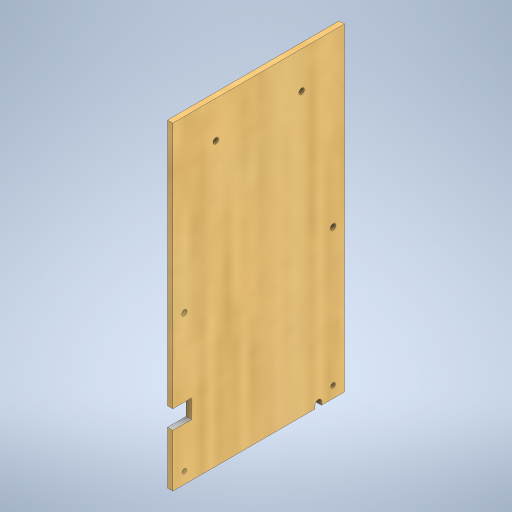
# Autodesk Inventor part: Panel2
Saved by Autodesk Inventor 2023 (Build 270158000, 158)
## iProperties
Created: 2022-12-03
Part Number: Panel2
Material: Genérico
Document SubType Name: Modeling
Designer: sergi
Density: 1 g/cm^3
Appearance: Valor por defecto
Author: sergi
Autodesk Inventor part; units mm, degrees
ref_plane "YZ Plane" through (0, 0, 0) normal (1, 0, 0) x (0, 1, 0)
ref_plane "XZ Plane" through (0, 0, 0) normal (0, 1, 0) x (-1, 0, 0)
ref_plane "XY Plane" through (0, 0, 0) normal (0, 0, 1) x (1, 0, 0)
sketch "Boceto1" plane through (0, 0, 0) normal (0, 1, 0) x (-1, 0, 0)
  line L0 (-1.5, -48.5) -> (1.5, -48.5)
  line L1 (1.5, -48.5) -> (1.5, 48.5)
  line L2 (1.5, 48.5) -> (-1.5, 48.5)
  line L3 (-1.5, 48.5) -> (-1.5, -48.5)
  line L4 (-1.5, -48.5) -> (1.5, 48.5) construction
  line L5 (1.5, -48.5) -> (-1.5, 48.5) construction
  point P0 (0, 0)
  dimension "d0" = 3
  dimension "d1" = 97
  constraints: 12 end point, 2 midpoint, 2 parallel, 1 horizontal, 1 perpendicular
  measures "d0" distance of L2.end L1.end
  measures "d1" distance of L1.end L0.end
extrude "Extrusión1" add sketch "Boceto1" along normal blind 180
sketch "Boceto2" plane through (-1.5, 0, -48.5) normal (-1, 0, 0) x (0, 0, 1)
  circle A0 centre (24.25, 159.25) radius 1.5 projected
  circle A1 centre (72.75, 159.25) radius 1.5 projected
  circle A2 centre (90.5, 84) radius 1.5 projected
  circle A3 centre (6.5, 84) radius 1.5 projected
  circle A4 centre (6.5, 6.5) radius 1.25 projected
  circle A5 centre (90.5, 6.5) radius 1.25 projected
  point P0 (48.5, 0)
extrude "Extrusión2" cut sketch "Boceto2" against normal through all
sketch "Boceto3" plane through (1.5, 0, 48.5) normal (1, 0, 0) x (0, 0, -1)
  line L0 (10.5, 26) -> (5.5, 26)
  line L1 (10.5, 44) -> (10.5, 26)
  line L2 (5.5, 44) -> (-0.0781, 44)
  line L3 (-0.0781, 26) -> (5.5, 26)
  line L4 (0, 0) -> (0, 180) projected
  line L5 (0, 44) -> (10.5, 44)
  line L6 (10.5, 44) -> (10.5, 26)
  line L7 (10.5, 26) -> (0, 26)
  line L8 (0, 26) -> (0, 44)
  line L9 (0, 35) -> (10.5, 35)
  line L10 (10.5, 29.75) -> (0, 29.75)
  line L11 (0, 29.75) -> (0, 40.25)
  line L12 (0, 40.25) -> (10.5, 40.25)
  line L13 (10.5, 40.25) -> (10.5, 29.75)
  line L14 (10.5, 29.75) -> (0, 40.25) construction
  line L15 (0, 29.75) -> (10.5, 40.25) construction
  point P0 (48.5, 0)
  point P1 (5.25, 35)
  point P2 (10.5, 40.25)
  point P3 (10.5, 29.75)
  dimension "d13" = 10.5
  constraints: 30 end point, 5 midpoint, 5 parallel, 4 horizontal, 3 point on line, 2 perpendicular
  measures "d13" distance of L10.end L11.end
extrude "Extrusión3" cut sketch "Boceto3" against normal through all contours L10 L4 L9 L1 | L9 L4 L12 L1
sketch "Boceto4" plane through (1.5, 0, 48.5) normal (1, 0, 0) x (0, 0, -1)
  line L0 (84, 0) -> (84, 13) projected
  line L1 (100, 0) -> (-3, 0) projected
  arc A0 (84, 1.85) -> (80.3, 1.85) centre (82.15, 1.85) ccw
  line L2 (0, 0) -> (97, 0) projected
  line L3 (80.3, 1.85) -> (80.3, 0)
  line L4 (97, 0) -> (0, 0) projected
  line L5 (84, 1.85) -> (84, 0)
  point P0 (48.5, 0)
  dimension "d9" = 3.7
  constraints: 4 end point, 3 tangent, 2 point on circle, 2 point on line, 1 centre point, 1 collinear, 1 perpendicular
  measures "d9" diameter of A0
extrude "Extrusión4" cut sketch "Boceto4" against normal through all
